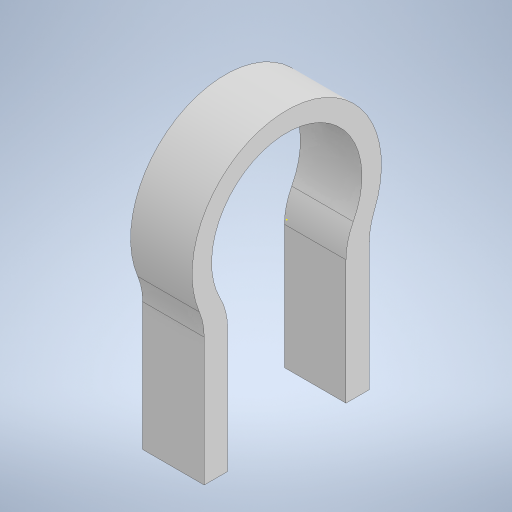
# Autodesk Inventor part: eye motor holder2
Saved by Autodesk Inventor 2024.3 (Build 283343010, 343A)
## iProperties
Created: 2025-04-07
Part Number: eye motor holder2
Material: Generic
Document SubType Name: Modeling
Designer: Vincent Larson
Density: 1 g/cm^3
Appearance: Default
Author: Vincent Larson
## iProperties of the stored document eye motor holder2_3DPrint.ipt
Created: 2025-04-08
Part Number: eye motor holder2_3DPrint
Material: Generic
Document SubType Name: Modeling
Designer: Vincent Larson
Density: 1 g/cm^3
Appearance: Default
Author: Vincent Larson
Autodesk Inventor part; units mm, degrees
ref_plane "YZ Plane" through (0, 0, 0) normal (1, 0, 0) x (0, 1, 0)
ref_plane "XZ Plane" through (0, 0, 0) normal (0, 1, 0) x (-1, 0, 0)
ref_plane "XY Plane" through (0, 0, 0) normal (0, 0, 1) x (1, 0, 0)
sketch "Sketch1" plane through (0, 0, 0) normal (1, 0, 0) x (0, 1, 0)
  line L0 (-7.458, 13.2905) -> (-7.458, -13.2905)
  arc A0 (-7.458, -9.5323) -> (-7.458, 9.5323) centre (0, 0) ccw
  arc A1 (-7.458, -13.2905) -> (-7.458, 13.2905) centre (0, 0) ccw
  point P0 (0, 0)
  constraints: 4 point on circle, 2 centre point, 2 end point, 2 point on line, 1 vertical
extrude "Extrusion1" add sketch "Sketch1" along normal blind 9.906 contours A1 L0 A0
sketch "Sketch2" plane through (0, -7.458, 9.5323) normal (0, -1, 0) x (1, 0, 0)
  line L0 (9.906, 3.7582) -> (9.906, 0) projected
  line L1 (9.906, 3.7582) -> (0, 3.7582)
  line L2 (0, 3.7582) -> (0, 0)
  line L3 (0, 0) -> (9.906, 0)
  line L4 (9.906, 0) -> (9.906, 3.7582)
  point P0 (0, -9.5323)
  constraints: 8 end point, 2 parallel, 1 horizontal, 1 perpendicular
extrude "Extrusion2" add sketch "Sketch2" along normal blind 22.9108
sketch "Sketch3" plane through (0, -7.458, -13.2905) normal (0, -1, 0) x (1, 0, 0)
  line L0 (9.906, 3.7582) -> (9.906, 0) projected
  line L1 (9.906, 3.7582) -> (0, 3.7582)
  line L2 (0, 3.7582) -> (0, 0)
  line L3 (0, 0) -> (9.906, 0)
  line L4 (9.906, 0) -> (9.906, 3.7582)
  point P0 (0, 13.2905)
  constraints: 8 end point, 2 parallel, 1 horizontal, 1 perpendicular
extrude "Extrusion3" add sketch "Sketch3" along normal blind 22.9108
fillet "Fillet1" radius 10.16 1 edges at (4.953, -7.458, -9.5323)
fillet "Fillet2" radius 10.16 1 edges at (4.953, -7.458, 9.5323)
fillet "Fillet3" radius 10.16 1 edges at (4.953, -7.458, 13.2905)
fillet "Fillet4" radius 10.16 1 edges at (4.953, -7.458, -13.2905)
sketch "Sketch5" plane through (9.906, 0, 0) normal (1, 0, 0) x (0, 0, -1)
  point P0 (0, 0)
body "Solid1"
